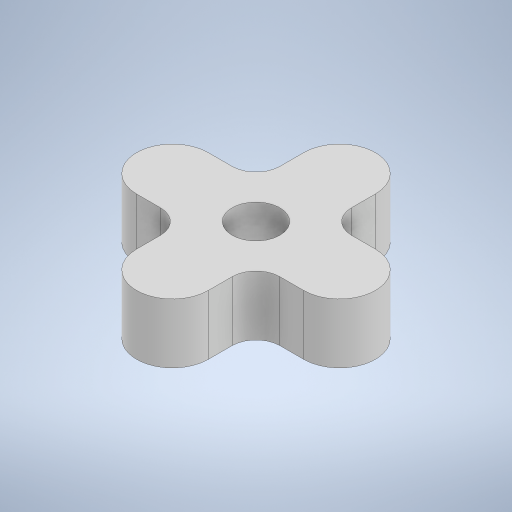
# Autodesk Inventor part: baterry
Saved by Autodesk Inventor 2024.1 (Build 281209000, 209)
## iProperties
Created: 2024-11-07
Part Number: baterry
Material: Všeobecné
Document SubType Name: Modeling
Designer: elias
Density: 1 g/cm^3
Appearance: Výchozí
Author: elias
Autodesk Inventor part; units mm, degrees
ref_plane "YZ Plane" through (0, 0, 0) normal (1, 0, 0) x (0, 1, 0)
ref_plane "XZ Plane" through (0, 0, 0) normal (0, 1, 0) x (-1, 0, 0)
ref_plane "XY Plane" through (0, 0, 0) normal (0, 0, 1) x (1, 0, 0)
sketch "Náčrt1" plane through (0, 0, 0) normal (0, 0, 1) x (1, 0, 0)
  circle A0 centre (0, 0) radius 2
  line L0 (0, -7) -> (0, 7) construction
  line L1 (3, 5) -> (3, 7)
  line L2 (-3, 7) -> (-3, 5)
  arc A1 (-3, -7) -> (3, -7) centre (0, -7) ccw
  arc A2 (3, 7) -> (-3, 7) centre (0, 7) ccw
  line L3 (-7, 0) -> (7, 0) construction
  line L4 (-7, -3) -> (-5, -3)
  line L5 (-5, 3) -> (-7, 3)
  arc A3 (-7, 3) -> (-7, -3) centre (-7, 0) ccw
  arc A4 (7, -3) -> (7, 3) centre (7, 0) ccw
  arc A5 (-5, 3) -> (-3, 5) centre (-5, 5) ccw
  line L6 (-3, -7) -> (-3, -5)
  line L7 (3, -7) -> (3, -5)
  line L8 (5, -3) -> (7, -3)
  line L9 (7, 3) -> (5, 3)
  line L10 (3, 7) -> (3, 3)
  arc A6 (-3, -5) -> (-5, -3) centre (-5, -5) ccw
  arc A7 (5, -3) -> (3, -5) centre (5, -5) ccw
  arc A8 (3, 5) -> (5, 3) centre (5, 5) ccw
  point P0 (3, -3)
  dimension "d0" = 4
  dimension "d1" = 7
  dimension "d2" = 6
  dimension "d3" = 7
  dimension "d4" = 6
  dimension "d5" = 2
  dimension "d6" = 2
  constraints: 26 end point, 16 point on circle, 16 tangent, 10 point on line, 9 centre point, 3 perpendicular, 2 equal radius, 2 midpoint, 2 parallel, 1 coincident, 1 collinear, 1 vertical
  measures "d0" diameter of A0
  measures "d1" distance of A0.centre L0.end
  measures "d2" diameter of A2
  measures "d3" distance of A0.centre L3.end
  measures "d4" diameter of A4
  measures "d5" radius of A5
  measures "d6" radius of A6
extrude "Vysunutí1" add sketch "Náčrt1" along normal blind 5
